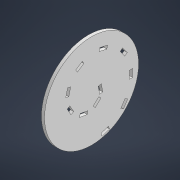
# Autodesk Inventor part: Стенка барабана
Saved by Autodesk Inventor 2022 (Build 260153000, 153)
## iProperties
Created: 2023-02-11
Part Number: Стенка барабана
Material: Типовые
Document SubType Name: Modeling
Designer: Глеб
Density: 1 g/cm^3
Appearance: По умолчанию
Author: Глеб
Autodesk Inventor part; units mm, degrees
ref_plane "YZ Plane" through (0, 0, 0) normal (1, 0, 0) x (0, 1, 0)
ref_plane "XZ Plane" through (0, 0, 0) normal (0, 1, 0) x (-1, 0, 0)
ref_plane "XY Plane" through (0, 0, 0) normal (0, 0, 1) x (1, 0, 0)
sketch "Эскиз1" plane through (0, 0, 0) normal (1, 0, 0) x (0, 1, 0)
  circle A0 centre (0, 0) radius 60
  point P0 (0, -60)
  constraints: 2 vertical alignment, 1 coincident, 4 other
extrude "Выдавливание1" add sketch "Эскиз1" along normal blind 4
sketch "Эскиз2" plane through (4, 0, 0) normal (1, 0, 0) x (0, 0, -1)
  point P0 (0, 0)
  point P1 (0, -60)
  constraints: 1 vertical alignment, 2 other
sketch "Эскиз3" plane through (4, 0, 0) normal (1, 0, 0) x (0, 0, -1)
  line L0 (0, -92.75) -> (0, 85.4583) construction
  circle A0 centre (0, 0) radius 60 construction
  line L1 (40.5908, -40.3227) -> (46.095, -31.9738)
  line L2 (46.095, -31.9738) -> (42.7554, -29.7722)
  line L3 (42.7554, -29.7722) -> (37.2513, -38.1211)
  line L4 (37.2513, -38.1211) -> (40.5908, -40.3227)
  line L5 (40.5908, -40.3227) -> (42.7554, -29.7722) construction
  line L6 (46.095, -31.9738) -> (37.2513, -38.1211) construction
  line L7 (41.6731, -35.0475) -> (44.4252, -30.873) construction
  line L8 (31.7471, -46.47) -> (48.2596, -21.4233) construction
  line L9 (48.2596, -21.4233) -> (51.5992, -23.6249) construction
  line L10 (51.5992, -23.6249) -> (35.0866, -48.6716) construction
  line L11 (35.0866, -48.6716) -> (31.7471, -46.47) construction
  line L12 (31.7471, -46.47) -> (51.5992, -23.6249) construction
  line L13 (48.2596, -21.4233) -> (35.0866, -48.6716) construction
  circle A1 centre (0, 0) radius 60 projected
  line L14 (48.3995, -11.3168) -> (48.3995, -1.3168)
  line L15 (48.3995, -1.3168) -> (52.3995, -1.3168)
  line L16 (52.3995, -1.3168) -> (52.3995, -11.3168) construction
  line L17 (52.3995, -11.3168) -> (48.3995, -11.3168)
  line L18 (48.3995, -11.3168) -> (52.3995, -1.3168) construction
  line L19 (48.3995, -1.3168) -> (52.3995, -11.3168) construction
  line L20 (48.3995, -21.3168) -> (48.3995, 8.6832) construction
  line L21 (48.3995, 8.6832) -> (52.3995, 8.6832) construction
  line L22 (52.3995, 8.6832) -> (52.3995, -21.3168)
  line L23 (52.3995, -21.3168) -> (48.3995, -21.3168) construction
  line L24 (48.3995, -21.3168) -> (52.3995, 8.6832) construction
  line L25 (48.3995, 8.6832) -> (52.3995, -21.3168) construction
  line L26 (50.3995, -6.3168) -> (50.3995, 8.6832) construction
  line L27 (36.4646, 25.3316) -> (42.4094, 17.2905)
  line L28 (42.4094, 17.2905) -> (45.6259, 19.6684)
  line L29 (45.6259, 19.6684) -> (39.6811, 27.7095)
  line L30 (39.6811, 27.7095) -> (36.4646, 25.3316)
  line L31 (36.4646, 25.3316) -> (45.6259, 19.6684) construction
  line L32 (42.4094, 17.2905) -> (39.6811, 27.7095) construction
  line L33 (30.5198, 33.3727) -> (48.3542, 9.2494) construction
  line L34 (48.3542, 9.2494) -> (51.5707, 11.6273) construction
  line L35 (51.5707, 11.6273) -> (33.7363, 35.7506) construction
  line L36 (33.7363, 35.7506) -> (30.5198, 33.3727) construction
  line L37 (30.5198, 33.3727) -> (51.5707, 11.6273) construction
  line L38 (48.3542, 9.2494) -> (33.7363, 35.7506) construction
  line L39 (41.0453, 22.5) -> (32.1281, 34.5617) construction
  line L40 (10.536, 42.571) -> (20.3099, 40.4564)
  line L41 (20.3099, 40.4564) -> (19.464, 36.5468)
  line L42 (19.464, 36.5468) -> (9.6901, 38.6615)
  line L43 (9.6901, 38.6615) -> (10.536, 42.571)
  line L44 (10.536, 42.571) -> (19.464, 36.5468) construction
  line L45 (20.3099, 40.4564) -> (9.6901, 38.6615) construction
  line L46 (-0.0837, 40.7762) -> (29.2378, 34.4321) construction
  line L47 (29.2378, 34.4321) -> (30.0837, 38.3417) construction
  line L48 (30.0837, 38.3417) -> (0.7622, 44.6857) construction
  line L49 (0.7622, 44.6857) -> (-0.0837, 40.7762) construction
  line L50 (-0.0837, 40.7762) -> (30.0837, 38.3417) construction
  line L51 (29.2378, 34.4321) -> (0.7622, 44.6857) construction
  line L52 (0.3392, 42.7309) -> (15, 39.5589) construction
  line L53 (-20.2765, 33.1516) -> (-11.9215, 38.6465)
  line L54 (-11.9215, 38.6465) -> (-9.7235, 35.3046)
  line L55 (-9.7235, 35.3046) -> (-18.0785, 29.8096)
  line L56 (-18.0785, 29.8096) -> (-20.2765, 33.1516)
  line L57 (-20.2765, 33.1516) -> (-9.7235, 35.3046) construction
  line L58 (-11.9215, 38.6465) -> (-18.0785, 29.8096) construction
  line L59 (-26.4334, 24.3146) -> (-1.3686, 40.7995) construction
  line L60 (-1.3686, 40.7995) -> (-3.5666, 44.1415) construction
  line L61 (-3.5666, 44.1415) -> (-28.6314, 27.6566) construction
  line L62 (-28.6314, 27.6566) -> (-26.4334, 24.3146) construction
  line L63 (-26.4334, 24.3146) -> (-3.5666, 44.1415) construction
  line L64 (-1.3686, 40.7995) -> (-28.6314, 27.6566) construction
  line L65 (-15, 34.2281) -> (-2.4676, 42.4705) construction
  line L66 (-32.897, 9.0632) -> (-30.5956, 18.7948)
  line L67 (-30.5956, 18.7948) -> (-26.703, 17.8742)
  line L68 (-26.703, 17.8742) -> (-29.0044, 8.1427)
  line L69 (-29.0044, 8.1427) -> (-32.897, 9.0632)
  line L70 (-32.897, 9.0632) -> (-26.703, 17.8742) construction
  line L71 (-30.5956, 18.7948) -> (-29.0044, 8.1427) construction
  line L72 (-34.0478, 4.1975) -> (-29.4449, 23.6606) construction
  line L73 (-29.4449, 23.6606) -> (-25.5522, 22.74) construction
  line L74 (-25.5522, 22.74) -> (-30.1551, 3.2769) construction
  line L75 (-30.1551, 3.2769) -> (-34.0478, 4.1975) construction
  line L76 (-34.0478, 4.1975) -> (-25.5522, 22.74) construction
  line L77 (-29.4449, 23.6606) -> (-30.1551, 3.2769) construction
  line L78 (-29.8, 13.4687) -> (-27.4986, 23.2003) construction
  line L79 (-30.1437, 1.6896) -> (-20.3668, -15.7578) construction
  line L80 (-20.3668, -15.7578) -> (-23.8563, -17.7132) construction
  line L81 (-23.8563, -17.7132) -> (-33.6332, -0.2658) construction
  line L82 (-33.6332, -0.2658) -> (-30.1437, 1.6896) construction
  line L83 (-30.1437, 1.6896) -> (-23.8563, -17.7132) construction
  line L84 (-20.3668, -15.7578) -> (-33.6332, -0.2658) construction
  line L85 (-27.6995, -2.6723) -> (-22.811, -11.396)
  line L86 (-22.811, -11.396) -> (-26.3005, -13.3514)
  line L87 (-26.3005, -13.3514) -> (-31.189, -4.6277)
  line L88 (-31.189, -4.6277) -> (-27.6995, -2.6723)
  line L89 (-27.6995, -2.6723) -> (-26.3005, -13.3514) construction
  line L90 (-22.811, -11.396) -> (-31.189, -4.6277) construction
  line L91 (-27, -8.0118) -> (-31.8884, 0.7119) construction
  line L92 (-19.4768, -16.8116) -> (0.1967, -20.411) construction
  line L93 (0.1967, -20.411) -> (-0.5232, -24.3456) construction
  line L94 (-0.5232, -24.3456) -> (-20.1967, -20.7463) construction
  line L95 (-20.1967, -20.7463) -> (-19.4768, -16.8116) construction
  line L96 (-19.4768, -16.8116) -> (-0.5232, -24.3456) construction
  line L97 (0.1967, -20.411) -> (-20.1967, -20.7463) construction
  line L98 (-14.5584, -17.7114) -> (-4.7217, -19.5111)
  line L99 (-4.7217, -19.5111) -> (-5.4416, -23.4458)
  line L100 (-5.4416, -23.4458) -> (-15.2783, -21.6461)
  line L101 (-15.2783, -21.6461) -> (-14.5584, -17.7114)
  line L102 (-14.5584, -17.7114) -> (-5.4416, -23.4458) construction
  line L103 (-4.7217, -19.5111) -> (-15.2783, -21.6461) construction
  line L104 (-10, -20.5786) -> (-19.8367, -18.7789) construction
  line L105 (11.0144, -9.2398) -> (0.2107, -19.6457) construction
  line L106 (0.2107, -19.6457) -> (2.9856, -22.5267) construction
  line L107 (2.9856, -22.5267) -> (13.7893, -12.1208) construction
  line L108 (13.7893, -12.1208) -> (11.0144, -9.2398) construction
  line L109 (11.0144, -9.2398) -> (2.9856, -22.5267) construction
  line L110 (0.2107, -19.6457) -> (13.7893, -12.1208) construction
  line L111 (9.2138, -10.9742) -> (2.0113, -17.9114)
  line L112 (2.0113, -17.9114) -> (4.7862, -20.7923)
  line L113 (4.7862, -20.7923) -> (11.9887, -13.8551)
  line L114 (11.9887, -13.8551) -> (9.2138, -10.9742)
  line L115 (9.2138, -10.9742) -> (4.7862, -20.7923) construction
  line L116 (2.0113, -17.9114) -> (11.9887, -13.8551) construction
  line L117 (7, -15.8832) -> (10.6012, -12.4146) construction
  line L118 (10.3281, -8.9147) -> (8.5366, 0.9236)
  line L119 (8.5366, 0.9236) -> (12.4719, 1.6401)
  line L120 (12.4719, 1.6401) -> (14.2634, -8.1981)
  line L121 (14.2634, -8.1981) -> (10.3281, -8.9147)
  line L122 (10.3281, -8.9147) -> (12.4719, 1.6401) construction
  line L123 (8.5366, 0.9236) -> (14.2634, -8.1981) construction
  line L124 (10.3281, -8.9147) -> (8.5366, 0.9236)
  line L125 (8.5366, 0.9236) -> (12.4719, 1.6401)
  line L126 (12.4719, 1.6401) -> (14.2634, -8.1981)
  line L127 (14.2634, -8.1981) -> (10.3281, -8.9147)
  line L128 (10.3281, -8.9147) -> (12.4719, 1.6401) construction
  line L129 (8.5366, 0.9236) -> (14.2634, -8.1981) construction
  line L130 (11.4, -3.6373) -> (10.5043, 1.2819) construction
  line L131 (-0.9405, 1.4271) -> (9.0554, 1.7143)
  line L132 (9.0554, 1.7143) -> (8.9405, 5.7126)
  line L133 (8.9405, 5.7126) -> (-1.0554, 5.4255)
  line L134 (-1.0554, 5.4255) -> (-0.9405, 1.4271)
  line L135 (-0.9405, 1.4271) -> (8.9405, 5.7126) construction
  line L136 (9.0554, 1.7143) -> (-1.0554, 5.4255) construction
  line L137 (-0.9405, 1.4271) -> (9.0554, 1.7143)
  line L138 (9.0554, 1.7143) -> (8.9405, 5.7126)
  line L139 (8.9405, 5.7126) -> (-1.0554, 5.4255)
  line L140 (-1.0554, 5.4255) -> (-0.9405, 1.4271)
  line L141 (-0.9405, 1.4271) -> (8.9405, 5.7126) construction
  line L142 (9.0554, 1.7143) -> (-1.0554, 5.4255) construction
  line L143 (4, 3.5699) -> (-0.9979, 3.4263) construction
  line L144 (3.8726, -59.8749) -> (32.3753, -50.5157) construction
  line L145 (32.3753, -50.5157) -> (31.1274, -46.7154) construction
  line L146 (31.1274, -46.7154) -> (2.6247, -56.0745) construction
  line L147 (2.6247, -56.0745) -> (3.8726, -59.8749) construction
  line L148 (3.8726, -59.8749) -> (31.1274, -46.7154) construction
  line L149 (32.3753, -50.5157) -> (2.6247, -56.0745) construction
  line L150 (13.3735, -56.7552) -> (22.8744, -53.6355)
  line L151 (22.8744, -53.6355) -> (21.6265, -49.8351)
  line L152 (21.6265, -49.8351) -> (12.1256, -52.9548)
  line L153 (12.1256, -52.9548) -> (13.3735, -56.7552)
  line L154 (13.3735, -56.7552) -> (21.6265, -49.8351) construction
  line L155 (22.8744, -53.6355) -> (12.1256, -52.9548) construction
  line L156 (17.5, -53.2951) -> (31.7514, -48.6155) construction
  point P0 (0, -60)
  point P1 (50.3995, -6.3168)
  point P2 (41.0453, 22.5)
  point P3 (15, 39.5589)
  point P4 (15, 39.5589)
  point P5 (-15, 34.2281)
  point P6 (-15, 34.2281)
  point P7 (-15, 34.2281)
  point P8 (-29.8, 13.4687)
  point P9 (-29.8, 13.4687)
  point P10 (-27, -8.0118)
  point P11 (-27, -8.0118)
  point P12 (-10, -20.5786)
  point P13 (7, -15.8832)
  point P14 (7, -15.8832)
  point P15 (11.4, -3.6373)
  point P16 (4, 3.5699)
  point P17 (4, 3.5699)
  point P18 (17.5, -53.2951)
  dimension "d83" = 0
  dimension "d84" = 1
  dimension "d93" = 10
  dimension "d94" = 4
  dimension "d95" = 30
  dimension "d96" = 10
  dimension "d98" = 4
  dimension "d99" = 30
  dimension "d100" = 10
  dimension "d101" = 30
  dimension "d102" = 4
  dimension "d103" = 22.5
  dimension "d104" = 10
  dimension "d105" = 30
  dimension "d106" = 4
  dimension "d107" = 15
  dimension "d108" = 30
  dimension "d109" = 4
  dimension "d110" = 10
  dimension "d111" = 15
  dimension "d112" = 10
  dimension "d113" = 20
  dimension "d114" = 4
  dimension "d115" = 29.8
  dimension "d116" = 20
  dimension "d117" = 10
  dimension "d118" = 4
  dimension "d119" = 27
  dimension "d120" = 10
  dimension "d121" = 20
  dimension "d122" = 4
  dimension "d123" = 10
  dimension "d124" = 10
  dimension "d125" = 15
  dimension "d127" = 4
  dimension "d128" = 7
  dimension "d132" = 10
  dimension "d134" = 4
  dimension "d135" = 10
  dimension "d136" = 11.4
  dimension "d137" = 10
  dimension "d138" = 10
  dimension "d139" = 4
  dimension "d140" = 4
  dimension "d141" = 4
  dimension "d142" = 30
  dimension "d143" = 10
  dimension "d144" = 17.5
  constraints: 312 end point, 84 midpoint, 55 parallel, 31 perpendicular, 9 collinear, 3 point on circle, 2 vertical, 1 coincident, 24 other
  measures "d93" distance of L1.start L1.end
  measures "d94" distance of L1.end L2.end
  measures "d95" distance of L9.end L10.end
  measures "d96" distance of L15.end L16.end
  measures "d98" distance of L20.end L21.end
  measures "d99" distance of L21.end L22.end
  measures "d100" distance of L28.end L29.end
  measures "d101" distance of L34.end L35.end
  measures "d102" distance of L35.end L33.start
  measures "d103" vertical distance of point (0, 0) point (41.045, 22.5)
  measures "d104" distance between parallel lines of L41 L43
  measures "d105" distance between parallel lines of L47 L49
  measures "d106" distance of L46.end L47.end
  measures "d107" horizontal distance of point (15, 39.559) point (0, 0)
  measures "d108" distance of L60.end L61.end
  measures "d109" distance of L53.end L54.end
  measures "d110" distance between parallel lines of L56 L54
  measures "d111" horizontal distance of point (-15, 34.228) point (0, 0)
  measures "d112" distance between parallel lines of L69 L67
  measures "d113" distance between parallel lines of L75 L73
  measures "d114" distance of L72.end L73.end
  measures "d115" horizontal distance of point (0, 0) point (-29.8, 13.469)
  measures "d116" distance of L79.start L79.end
  measures "d117" distance of L85.start L85.end
  measures "d118" distance of L79.end L80.end
  measures "d119" horizontal distance of point (0, 0) point (-27, -8.012)
  measures "d120" distance between parallel lines of L99 L101
  measures "d121" distance between parallel lines of L95 L93
  measures "d122" distance of L92.end L93.end
  measures "d123" horizontal distance of point (0, 0) point (-10, -20.579)
  measures "d124" distance between parallel lines of L112 L114
  measures "d125" distance of L106.end L107.end
  measures "d127" distance of L107.end L105.start
  measures "d128" horizontal distance of point (0, 0) point (7, -15.883)
  measures "d132" distance of L125.end L126.end
  measures "d134" distance of L124.end L125.end
  measures "d135" distance between parallel lines of L121 L119
  measures "d136" horizontal distance of point (0, 0) L130.start
  measures "d137" distance between parallel lines of L138 L140
  measures "d138" distance between parallel lines of L132 L134
  measures "d139" distance of L131.end L132.end
  measures "d140" horizontal distance of point (0, 0) point (4, 3.57)
  measures "d141" distance of L146.end L144.start
  measures "d142" distance of L145.end L146.end
  measures "d143" distance between parallel lines of L151 L153
  measures "d144" distance from line of L0 point (17.5, -53.295)
extrude "Выдавливание2" cut sketch "Эскиз3" against normal through all contours L4 L3 L2 L1 | L14 L15 L22 L17 | L30 L29 L28 L27 | L40 L41 L42 L43 | L53 L54 L55 L56 | L66 L67 L68 L69 | L85 L86 L87 L88 | L98 L99 L100 L101 | L114 L113 L112 L111 | L118 L119 L120 L121 | L153 L152 L151 L150
